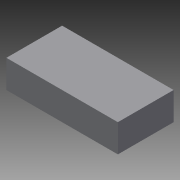
# Autodesk Inventor part: wozek
Saved by Autodesk Inventor 2014 (Build 180170000, 170)
## iProperties
Created: 2013-12-25
Part Number: wozek
Material: Ogólny
Document SubType Name: Modeling
Designer: Kuba
Density: 1 g/cm^3
Appearance: Domyślna
Author: Kuba
Autodesk Inventor part; units mm, degrees
ref_plane "YZ Plane" through (0, 0, 0) normal (1, 0, 0) x (0, 1, 0)
ref_plane "XZ Plane" through (0, 0, 0) normal (0, 1, 0) x (-1, 0, 0)
ref_plane "XY Plane" through (0, 0, 0) normal (0, 0, 1) x (1, 0, 0)
sketch "Szkic1" plane through (0, 0, 0) normal (1, 0, 0) x (0, 1, 0)
  line L0 (-38, 45.5) -> (-9, 45.5)
  line L1 (-9, 45.5) -> (-9, 25.5)
  line L2 (-9, 25.5) -> (-38, 25.5)
  line L3 (-38, 25.5) -> (-38, 45.5)
  line L4 (-38, 45.5) -> (-9, 25.5) construction
  line L5 (-9, 45.5) -> (-38, 25.5) construction
  point P0 (0, 0)
  point P1 (-23.5, 35.5)
  dimension "d0" = 29
  dimension "d1" = 20
  constraints: 12 end point, 2 midpoint, 2 parallel, 1 horizontal, 1 perpendicular
  measures "d0" distance of L1.end L2.end
  measures "d1" distance of L0.end L1.end
extrude "Wyciągnięcie proste1" add sketch "Szkic1" along normal blind 70
fillet "Zaokrąglenie1" radius 0.5 2 edges at (35, -38, 25.5) (35, -9, 25.5)
